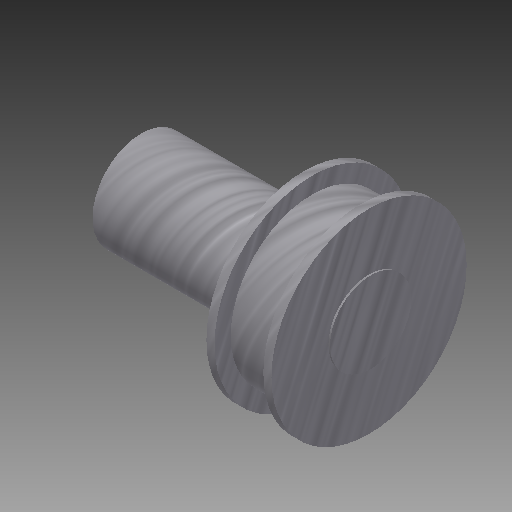
# Autodesk Inventor part: Roller2
Saved by Autodesk Inventor 2019 (Build 230136000, 136)
## iProperties
Created: 2017-01-18
Part Number: Roller2
Document SubType Name: Modeling
Designer: Administrator
Density: 1 g/cm^3
Mass: 0.633424 g
Surface Area: 6.17323 cm^2
Volume: 0.633424 cm^3
Material: Generic
Appearance: Aluminum (Machined)
Author: Administrator
Autodesk Inventor part; units mm, degrees
ref_plane "YZ Plane" through (0, 0, 0) normal (1, 0, 0) x (0, 1, 0)
ref_plane "XZ Plane" through (0, 0, 0) normal (0, 1, 0) x (-1, 0, 0)
ref_plane "XY Plane" through (0, 0, 0) normal (0, 0, 1) x (1, 0, 0)
sketch "Sketch1" plane through (0, 0, 0) normal (0, 0, 1) x (1, 0, 0)
  line L0 (0, 0) -> (0, 3)
  line L1 (0, 3) -> (10, 3)
  line L2 (10, 3) -> (10, 6)
  line L3 (10, 6) -> (10.5, 6)
  line L4 (10.5, 6) -> (10.5, 5)
  line L5 (10.5, 5) -> (13.5, 5)
  line L6 (13.5, 5) -> (13.5, 6)
  line L7 (13.5, 6) -> (14, 6)
  line L8 (14, 6) -> (14, 0)
  line L9 (14, 0) -> (0, 0)
  dimension "d0" = 3
  dimension "d1" = 10
  dimension "d2" = 0.5
  dimension "d3" = 5
  dimension "d4" = 0.5
  dimension "d5" = 1
  dimension "d6" = 3
  constraints: 20 end point, 9 parallel, 1 perpendicular, 1 vertical, 1 other
  measures "d0" distance between parallel lines of L1 L9
  measures "d1" distance between parallel lines of L0 L2
  measures "d2" distance of L2.end L3.end
  measures "d3" distance between parallel lines of L5 L9
  measures "d4" distance of L6.end L7.end
  measures "d5" distance between parallel lines of L3 L5
  measures "d6" distance of L4.end L5.end
revolve "Revolution1" add sketch "Sketch1" angle 360 about axis through (14, 0, 0) along (-1, 0, 0)
sketch "Sketch4" plane through (14, 0, 0) normal (1, 0, 0) x (0, 0, -1)
  circle A0 centre (0, 0) radius 6 projected
  circle A1 centre (0, 0) radius 2.5
  dimension "d22" = 5
  constraints: 1 centre point, 1 coincident
  measures "d22" diameter of A1
extrude "Extrusion2" add sketch "Sketch4" along normal blind 0.1 contours A1
body "Solid1"
